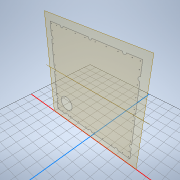
# Autodesk Inventor part: glas
Saved by Autodesk Inventor 2021 (Build 250183000, 183)
## iProperties
Created: 2021-06-22
Part Number: glas
Material: Tworzywo, przezroczyste
Document SubType Name: Modeling
Designer: Wojciech Wołczek
Density: 1.188 g/cm^3
Appearance: Przezroczyste — przejrzyste
Author: Wojciech Wołczek
Autodesk Inventor part; units mm, degrees
ref_plane "YZ Plane" through (0, 0, 0) normal (1, 0, 0) x (0, 1, 0)
ref_plane "XZ Plane" through (0, 0, 0) normal (0, 1, 0) x (-1, 0, 0)
ref_plane "XY Plane" through (0, 0, 0) normal (0, 0, 1) x (1, 0, 0)
ref_plane "Płaszczyzna konstrukcyjna1" through (0, 0, 0) normal (0, 0, 1) x (1, 0, 0)
sketch "Szkic1" plane through (0, 0, 0) normal (0, 0, 1) x (1, 0, 0)
  circle A0 centre (-437.5, -300) radius 4 projected
  circle A1 centre (-437.5, 300) radius 4 projected
  circle A2 centre (-300, 437.5) radius 4 projected
  circle A3 centre (300, 437.5) radius 4 projected
  circle A4 centre (437.5, 300) radius 4 projected
  circle A5 centre (437.5, -300) radius 4 projected
  circle A6 centre (-437.5, 0) radius 4 projected
  circle A7 centre (0, 437.5) radius 4 projected
  circle A8 centre (437.5, 0) radius 4 projected
  circle A9 centre (300, -437.5) radius 4 projected
  circle A10 centre (-300, -437.5) radius 4 projected
  circle A11 centre (0, -437.5) radius 4 projected
  line L0 (398.5, -398.5) -> (398.5, 398.5) projected
  line L1 (-398.5, -398.5) -> (398.5, -398.5) projected
  line L2 (-398.5, 398.5) -> (-398.5, -398.5) projected
  line L3 (398.5, 398.5) -> (-398.5, 398.5) projected
  line L4 (-457.5, -457.5) -> (-457.5, 457.5) projected
  line L5 (457.5, -457.5) -> (-457.5, -457.5) projected
  line L6 (457.5, 457.5) -> (457.5, -457.5) projected
  line L7 (-457.5, 457.5) -> (457.5, 457.5) projected
  line L8 (437.5, -437.5) -> (-437.5, -437.5)
  line L9 (-437.5, -437.5) -> (-437.5, 437.5)
  line L10 (-437.5, 437.5) -> (437.5, 437.5)
  line L11 (437.5, 437.5) -> (437.5, -437.5)
  line L12 (437.5, -437.5) -> (-437.5, 437.5) construction
  line L13 (-437.5, -437.5) -> (437.5, 437.5) construction
  circle A12 centre (-437.5, 300) radius 17.5
  circle A13 centre (-437.5, 0) radius 17.5
  circle A14 centre (-437.5, -300) radius 17.5
  circle A15 centre (-422.5, 422.5) radius 3
  circle A16 centre (-422.5, 362.5) radius 3
  circle A17 centre (-422.5, 250) radius 3
  circle A18 centre (-422.5, 150) radius 3
  circle A19 centre (-422.5, 50) radius 3
  line L14 (-437.5, 0) -> (437.5, 0) construction
  circle A20 centre (-422.5, -362.5) radius 3
  circle A21 centre (-422.5, -250) radius 3
  circle A22 centre (-422.5, -150) radius 3
  circle A23 centre (-422.5, -50) radius 3
  circle A24 centre (0, -437.5) radius 17.5
  circle A25 centre (-50, -422.5) radius 3
  circle A26 centre (-250, -422.5) radius 3
  line L15 (437.5, -437.5) -> (-437.5, -437.5)
  line L16 (0, -437.5) -> (0, 437.5) construction
  line L17 (437.5, 437.5) -> (-437.5, -437.5) construction
  circle A27 centre (50, -422.5) radius 3
  circle A28 centre (-150, -422.5) radius 3
  circle A29 centre (-422.5, -422.5) radius 3
  circle A30 centre (250, -422.5) radius 3
  circle A31 centre (362.5, -422.5) radius 3
  circle A32 centre (-362.5, -422.5) radius 3
  circle A33 centre (-300, -437.5) radius 17.5
  circle A34 centre (300, -437.5) radius 17.5
  circle A35 centre (150, -422.5) radius 3
  circle A36 centre (437.5, 0) radius 17.5
  circle A37 centre (422.5, -50) radius 3
  circle A38 centre (422.5, -250) radius 3
  line L18 (437.5, 437.5) -> (437.5, -437.5)
  line L19 (437.5, 0) -> (-437.5, 0) construction
  line L20 (-437.5, 437.5) -> (437.5, -437.5) construction
  circle A39 centre (422.5, 50) radius 3
  circle A40 centre (422.5, -150) radius 3
  circle A41 centre (422.5, -422.5) radius 3
  circle A42 centre (422.5, 250) radius 3
  circle A43 centre (422.5, 362.5) radius 3
  circle A44 centre (422.5, -362.5) radius 3
  circle A45 centre (437.5, -300) radius 17.5
  circle A46 centre (437.5, 300) radius 17.5
  circle A47 centre (422.5, 150) radius 3
  circle A48 centre (0, 437.5) radius 17.5
  circle A49 centre (50, 422.5) radius 3
  circle A50 centre (250, 422.5) radius 3
  line L21 (-437.5, 437.5) -> (437.5, 437.5)
  line L22 (0, 437.5) -> (0, -437.5) construction
  line L23 (-437.5, -437.5) -> (437.5, 437.5) construction
  circle A51 centre (-50, 422.5) radius 3
  circle A52 centre (150, 422.5) radius 3
  circle A53 centre (422.5, 422.5) radius 3
  circle A54 centre (-250, 422.5) radius 3
  circle A55 centre (-362.5, 422.5) radius 3
  circle A56 centre (362.5, 422.5) radius 3
  circle A57 centre (300, 437.5) radius 17.5
  circle A58 centre (-300, 437.5) radius 17.5
  circle A59 centre (-150, 422.5) radius 3
  circle A60 centre (-362.5, 422.5) radius 3 projected
  circle A61 centre (50, 422.5) radius 3 projected
  circle A62 centre (422.5, 422.5) radius 3 projected
  circle A63 centre (422.5, 50) radius 3 projected
  circle A64 centre (422.5, -362.5) radius 3 projected
  circle A65 centre (150, -422.5) radius 3 projected
  circle A66 centre (-250, -422.5) radius 3 projected
  circle A67 centre (-422.5, -250) radius 3 projected
  circle A68 centre (-422.5, 150) radius 3 projected
  circle A69 centre (-422.5, 50) radius 3 projected
  circle A70 centre (-422.5, -362.5) radius 3 projected
  circle A71 centre (-150, -422.5) radius 3 projected
  circle A72 centre (250, -422.5) radius 3 projected
  circle A73 centre (422.5, -250) radius 3 projected
  circle A74 centre (422.5, 150) radius 3 projected
  circle A75 centre (362.5, 422.5) radius 3 projected
  circle A76 centre (-50, 422.5) radius 3 projected
  circle A77 centre (-422.5, 422.5) radius 3 projected
  circle A78 centre (-250, 422.5) radius 3 projected
  circle A79 centre (150, 422.5) radius 3 projected
  circle A80 centre (422.5, 362.5) radius 3 projected
  circle A81 centre (422.5, -50) radius 3 projected
  circle A82 centre (422.5, -422.5) radius 3 projected
  circle A83 centre (50, -422.5) radius 3 projected
  circle A84 centre (-362.5, -422.5) radius 3 projected
  circle A85 centre (-422.5, -150) radius 3 projected
  circle A86 centre (-422.5, 250) radius 3 projected
  circle A87 centre (-422.5, -50) radius 3 projected
  circle A88 centre (-422.5, -422.5) radius 3 projected
  circle A89 centre (-50, -422.5) radius 3 projected
  circle A90 centre (362.5, -422.5) radius 3 projected
  circle A91 centre (422.5, -150) radius 3 projected
  circle A92 centre (422.5, 250) radius 3 projected
  circle A93 centre (250, 422.5) radius 3 projected
  circle A94 centre (-150, 422.5) radius 3 projected
  circle A95 centre (-422.5, 362.5) radius 3 projected
  point P0 (0, 0)
  point P1 (0, 0)
  point P2 (0, 0)
  point P3 (0, 0)
  point P4 (-282.5, 437.5)
  point P5 (-317.5, 437.5)
  point P6 (-437.5, 317.5)
  point P7 (-437.5, 282.5)
  point P8 (-437.5, 17.5)
  point P9 (-437.5, -17.5)
  point P10 (-437.5, -282.5)
  point P11 (-437.5, -317.5)
  point P12 (-317.5, -437.5)
  point P13 (-282.5, -437.5)
  point P14 (-17.5, -437.5)
  point P15 (17.5, -437.5)
  point P16 (282.5, -437.5)
  point P17 (317.5, -437.5)
  point P18 (437.5, -317.5)
  point P19 (437.5, -282.5)
  point P20 (437.5, -17.5)
  point P21 (437.5, 17.5)
  point P22 (437.5, 282.5)
  point P23 (437.5, 317.5)
  point P24 (317.5, 437.5)
  point P25 (282.5, 437.5)
  point P26 (17.5, 437.5)
  point P27 (-17.5, 437.5)
  dimension "d0" = 875
  dimension "d1" = 35
  dimension "d4" = 300
  dimension "d9" = 6
  dimension "d10" = 15
  dimension "d11" = 6
  dimension "d12" = 15
  dimension "d13" = 60
  dimension "d14" = 6
  dimension "d15" = 6
  dimension "d16" = 6
  dimension "d17" = 100
  dimension "d18" = 100
  dimension "d19" = 15
  dimension "d20" = 15
  dimension "d21" = 15
  dimension "d22" = 50
  dimension "d25" = 360
  constraints: 48 centre point, 32 end point, 5 midpoint, 4 point on line, 4 symmetric about line, 3 coincident, 2 parallel, 1 horizontal, 1 perpendicular, 1 vertical, 135 other
  measures "d0" distance of L8.end L9.end
  measures "d1" diameter of A12
  measures "d4" distance of A12.centre L14.start
  measures "d9" diameter of A15
  measures "d10" distance from line of L9 A15.centre
  measures "d11" diameter of A16
  measures "d12" distance from line of L9 A16.centre
  measures "d13" distance of A15.centre A16.centre
  measures "d14" diameter of A17
  measures "d15" diameter of A18
  measures "d16" diameter of A19
  measures "d17" distance of A18.centre A19.centre
  measures "d18" distance of A17.centre A18.centre
  measures "d19" distance from line of L9 A17.centre
  measures "d20" distance from line of L9 A18.centre
  measures "d21" distance from line of L9 A19.centre
  measures "d22" vertical distance of A12.centre A17.centre
extrude "Wyciągnięcie proste1" add sketch "Szkic1" along normal blind 3 contours L9 A13 A12 L10 A58 A48 A57 L11 A46 A36 A45 L8 A34 A24 A33 A14 | L1 L2 L3 L0
sketch "Szkic2" plane through (0, 0, 3) normal (0, 0, 1) x (1, 0, 0)
  circle A0 centre (-300, -300) radius 75
  point P0 (0, 0)
  dimension "d29" = 150
  dimension "d30" = 300
  dimension "d31" = 300
  constraints: 1 centre point
  measures "d29" diameter of A0
  measures "d30" horizontal distance of point (0, 0) A0.centre
  measures "d31" horizontal distance of point (0, 0) A0.centre
extrude "Wyciągnięcie proste2" cut sketch "Szkic2" against normal blind 3
